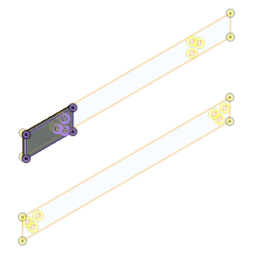
Chassis frame v1-1 (Autodesk Fusion 360 design; units mm, degrees)
Autodesk Fusion 360 part; units mm, degrees
sketch "Design sketch" plane through (0, 0, 0) normal (1, 0, 0) x (0, 1, 0)
  line L0 (100, 10) -> (-100, 10)
  line L1 (-100, 10) -> (-100, -10)
  line L2 (-100, -10) -> (100, -10)
  line L3 (100, -10) -> (100, 10)
  line L4 (100, 10) -> (-100, -10) construction
  line L5 (-100, 10) -> (100, -10) construction
  circle A0 centre (-95, 3.5) radius 1.75
  circle A1 centre (-90, -3.5) radius 1.75
  circle A2 centre (-85, 3.5) radius 1.75
  circle A3 centre (-69.3758, 70) radius 1.75
  circle A4 centre (63.6242, 65) radius 1.75
  circle A5 centre (-62.3758, 75) radius 1.75
  line L6 (-99.3758, 80) -> (100.6242, 60) construction
  line L7 (100.6242, 80) -> (-99.3758, 80)
  line L8 (-99.3758, 80) -> (-99.3758, 60)
  line L9 (100.6242, 60) -> (100.6242, 80)
  circle A6 centre (-62.3758, 65) radius 1.75
  line L10 (-99.3758, 60) -> (100.6242, 60)
  circle A7 centre (70.6242, 70) radius 1.75
  circle A8 centre (63.6242, 75) radius 1.75
  line L11 (100.6242, 80) -> (-99.3758, 60) construction
  circle A9 centre (90, -3.5) radius 1.75
  circle A10 centre (95, 3.5) radius 1.75
  circle A11 centre (85, 3.5) radius 1.75
  line L12 (100.6242, 80) -> (-99.3758, 80)
  line L13 (-54.3758, 80) -> (-54.3758, 60)
  point P0 (0.6242, 70)
  point P1 (0.6242, 70)
  dimension "d1" = 200
  dimension "d2" = 20
  dimension "d5" = 3.5
  dimension "d8" = 3.5
  dimension "d9" = 3.5
  dimension "d26" = 200
  dimension "d27" = 20
  dimension "d28" = 3.5
  dimension "d29" = 70
  dimension "d30" = 3.5
  dimension "d31" = 3.5
  dimension "d32" = 7
  dimension "d33" = 5
  dimension "d34" = 5
  dimension "d35" = 3.5
  dimension "d36" = 3.5
  dimension "d37" = 3.5
  dimension "d38" = 5
  dimension "d39" = 5
  dimension "d40" = 7
  dimension "d41" = 70
  dimension "d43" = 7
  dimension "d44" = 5
  dimension "d45" = 5
  dimension "d46" = 90
  dimension "d47" = 3.5
  dimension "d48" = 3.5
  dimension "d49" = 3.5
  dimension "d50" = 3.5
  dimension "d51" = 7
  dimension "d52" = 5
  dimension "d53" = 5
  dimension "d54" = 90
  dimension "d55" = 3.5
  dimension "d69" = 55
  constraint horizontal L0
  constraint perpendicular L0 L1
  constraint parallel L0 L2
  constraint parallel L1 L3
  constraint coincident L4 origin
  constraint coincident L5 origin
  constraint horizontal L7
  constraint perpendicular L7 L8
  constraint parallel L7 L10
  constraint parallel L8 L9
  constraint coincident P1 L11
  constraint coincident P1 L6
  constraint coincident P1 P0
  constraint vertical A4.centre A8.centre
  constraint vertical A6.centre A5.centre
  constraint horizontal A0.centre A2.centre
  constraint horizontal A11.centre A10.centre
  constraint horizontal L12
  constraint coincident L7 L13.start
  constraint coincident L10 L13.end
  constraint perpendicular L10 L13
  measures "d1" distance of L1.end L2.end
  measures "d2" distance of L0.end L1.end
  measures "d5" diameter of A0
  measures "d8" diameter of A1
  measures "d9" diameter of A2
  measures "d26" distance of L8.end L6.end
  measures "d27" distance of L8.end L6.start
  measures "d28" diameter of A3
  measures "d29" distance of P1 A3.centre
  measures "d30" diameter of A6
  measures "d31" diameter of A5
  measures "d32" horizontal distance of A3.centre A5.centre
  measures "d33" vertical distance of A3.centre A5.centre
  measures "d34" vertical distance of A3.centre A6.centre
  measures "d35" diameter of A7
  measures "d36" diameter of A4
  measures "d37" diameter of A8
  measures "d38" vertical distance of A7.centre A8.centre
  measures "d39" vertical distance of A7.centre A4.centre
  measures "d40" horizontal distance of A7.centre A8.centre
  measures "d41" distance of P1 A7.centre
  measures "d43" vertical distance of A0.centre A1.centre
  measures "d44" horizontal distance of A0.centre A1.centre
  measures "d45" horizontal distance of A1.centre A2.centre
  measures "d46" horizontal distance of origin A1.centre
  measures "d47" vertical distance of origin A1.centre
  measures "d48" diameter of A11
  measures "d49" diameter of A9
  measures "d50" diameter of A10
  measures "d51" vertical distance of A11.centre A9.centre
  measures "d52" horizontal distance of A11.centre A9.centre
  measures "d53" horizontal distance of A9.centre A10.centre
  measures "d54" horizontal distance of origin A9.centre
  measures "d55" vertical distance of origin A9.centre
  measures "d69" distance of P1 L13
sketch "Laser cut ready sketch" plane through (0, 0, 0) normal (1, 0, 0) x (0, 1, 0)
  circle A0 centre (-69.3758, 70) radius 1.75
  circle A1 centre (63.6242, 65) radius 1.75
  circle A2 centre (-62.3758, 75) radius 1.75
  circle A3 centre (63.6242, 75) radius 1.75
  circle A4 centre (-62.3758, 65) radius 1.75
  circle A5 centre (70.6242, 70) radius 1.75
  line L0 (-99.3758, 80) -> (-99.3758, 60)
  line L1 (100.6242, 80) -> (-99.3758, 80)
  line L2 (100.6242, 60) -> (100.6242, 80)
  line L3 (-99.3758, 60) -> (100.6242, 60)
  circle A6 centre (-85, 3.5) radius 1.75
  circle A7 centre (85, 3.5) radius 1.75
  circle A8 centre (95, 3.5) radius 1.75
  circle A9 centre (90, -3.5) radius 1.75
  circle A10 centre (-95, 3.5) radius 1.75
  circle A11 centre (-90, -3.5) radius 1.75
  line L4 (-100, -10) -> (100, -10)
  line L5 (-100, 10) -> (-100, -10)
  line L6 (100, 10) -> (-100, 10)
  line L7 (100, -10) -> (100, 10)
extrude "Extrude6" add sketch "Design sketch" along normal blind 3 contours L7 L8 L10 L12 L13
sketch "Motor connector laser cur sketch" plane through (3, 0, 0) normal (1, 0, 0) x (0, 1, 0)
  circle A0 centre (-69.3758, 70) radius 1.75
  circle A1 centre (-62.3758, 75) radius 1.75
  circle A2 centre (-62.3758, 65) radius 1.75
  line L0 (-99.3758, 80) -> (-99.3758, 60)
  line L1 (-99.3758, 60) -> (-54.3758, 60)
  line L2 (-54.3758, 60) -> (-54.3758, 80)
  line L3 (-54.3758, 80) -> (-99.3758, 80)
  circle A3 centre (-62.3758, 65) radius 1.75
  circle A4 centre (-62.3758, 75) radius 1.75
  circle A5 centre (-69.3758, 70) radius 1.75
  line L4 (-54.3758, 80) -> (-99.3758, 80)
  line L5 (-54.3758, 80) -> (-54.3758, 60)
  line L6 (-99.3758, 60) -> (-54.3758, 60)
  line L7 (-99.3758, 80) -> (-99.3758, 60)
extrude "Extrude5" [suppressed]
extrude "Extrude2" [suppressed]
equation "d1 = width"
equation "d2 = partWidth"
equation "width = 200 mm"
equation "partWidth = 20 mm"
equation "d5 = boltHole"
equation "boltHole = 3.5 mm"
equation "d8 = boltHole"
equation "d9 = boltHole"
equation "boltTriangleHeight = 7 mm"
equation "boltTriangleWidthHalf = 5 mm"
equation "boltTriangleLongGapFromCenter = 90 mm"
equation "d26 = width"
equation "d27 = partWidth"
equation "d28 = boltHole"
equation "d29 = boltTriangleShortGapFromCenter"
equation "d30 = boltHole"
equation "d31 = boltHole"
equation "d32 = boltTriangleHeight"
equation "d33 = boltTriangleWidthHalf"
equation "d34 = boltTriangleWidthHalf"
equation "d35 = boltHole"
equation "d36 = boltHole"
equation "d37 = boltHole"
equation "d38 = boltTriangleWidthHalf"
equation "d39 = boltTriangleWidthHalf"
equation "d40 = boltTriangleHeight"
equation "d41 = boltTriangleShortGapFromCenter"
equation "boltTriangleShortGapFromCenter = 70 mm"
equation "d43 = boltTriangleHeight"
equation "d44 = boltTriangleWidthHalf"
equation "d45 = boltTriangleWidthHalf"
equation "d46 = boltTriangleLongGapFromCenter"
equation "d47 = boltTriangleHeight / 2"
equation "d48 = boltHole"
equation "d49 = boltHole"
equation "d50 = boltHole"
equation "d51 = boltTriangleHeight"
equation "d52 = boltTriangleWidthHalf"
equation "d53 = boltTriangleWidthHalf"
equation "d54 = boltTriangleLongGapFromCenter"
equation "d55 = boltTriangleHeight / 2"
